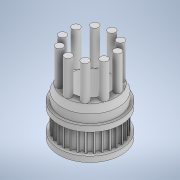
# Autodesk Inventor part: piece_roue_test_8
Saved by Autodesk Inventor 2020.1 (Build 241239000, 239)
## iProperties
Created: 2019-07-25
Part Number: piece_roue_test_8
Material: Générique
Document SubType Name: Modeling
Designer: marlo
Density: 1 g/cm^3
Appearance: Par défaut
Author: marlo
Autodesk Inventor part; units mm, degrees
ref_plane "YZ Plane" through (0, 0, 0) normal (1, 0, 0) x (0, 1, 0)
ref_plane "XZ Plane" through (0, 0, 0) normal (0, 1, 0) x (-1, 0, 0)
ref_plane "XY Plane" through (0, 0, 0) normal (0, 0, 1) x (1, 0, 0)
sketch "Esquisse2" plane through (0, 0, 0) normal (0, 1, 0) x (-1, 0, 0)
  circle A0 centre (0, 0) radius 18.5
  circle A1 centre (0, 0) radius 13.1
  dimension "d0" = 37
  dimension "d1" = 26.2
  constraints: 2 centre point, 2 coincident
  measures "d0" diameter of A0
  measures "d1" diameter of A1
extrude "Extrusion1" add sketch "Esquisse2" against normal blind 13
sketch "Esquisse3" plane through (0, 0, 0) normal (0, 1, 0) x (1, 0, 0)
  circle A0 centre (0, -15.8) radius 2.7
  line L0 (-22, 0) -> (25, 0) construction
  line L1 (-20, -18.5) -> (14, -18.5) construction
  circle A1 centre (0, 0) radius 18.5 construction
  circle A2 centre (-15.0267, 4.8825) radius 2.7
  line L2 (0, -15.8) -> (0, 0) construction
  line L3 (-15.0267, 4.8825) -> (0, 0) construction
  circle A3 centre (-15.0267, -4.8825) radius 2.7
  line L4 (0, 0) -> (-15.0267, -4.8825) construction
  line L5 (-15.0267, -4.8825) -> (-15.0267, 4.8825) construction
  line L6 (0, -31) -> (0, 24) construction
  line L7 (-15.0267, -4.8825) -> (-15.0267, -7.5825) construction
  line L8 (-15.0267, 4.8825) -> (-16.4693, 2.6002) construction
  line L9 (0, -15.8) -> (-2.3383, -17.15) construction
  circle A4 centre (-9.287, 12.7825) radius 2.7
  line L10 (0, 0) -> (-9.287, 12.7825) construction
  line L11 (-9.287, 12.7825) -> (-15.0267, 4.8825) construction
  line L12 (-9.287, 12.7825) -> (-7.7, 14.9668) construction
  circle A5 centre (-9.287, -12.7825) radius 2.7
  line L13 (-9.287, -12.7825) -> (0, 0) construction
  line L14 (-9.287, -12.7825) -> (0, -15.8) construction
  line L15 (-9.287, -12.7825) -> (-11.2119, -10.8891) construction
  line L16 (-9.287, -12.7825) -> (-15.0267, -4.8825) construction
  circle A6 centre (0, 15.8) radius 2.7
  line L17 (0, 15.8) -> (-1.5986, 17.9759) construction
  line L18 (0, 15.8) -> (0, 0) construction
  line L19 (0, 15.8) -> (-9.287, 12.7825) construction
  circle A7 centre (15.0267, 4.8825) radius 2.7
  circle A8 centre (15.0267, -4.8825) radius 2.7
  circle A9 centre (9.287, 12.7825) radius 2.7
  circle A10 centre (9.287, -12.7825) radius 2.7
  dimension "d4" = 5.4
  constraints: 40 end point, 14 equal length, 4 centre point, 4 symmetric about line, 3 horizontal, 3 point on line, 3 vertical, 1 coincident, 1 tangent, 1 vertical alignment, 21 other
extrude "Extrusion2" add sketch "Esquisse3" along normal blind 25
sketch "Esquisse4" plane through (0, -13, 0) normal (0, -1, 0) x (1, 0, 0)
  circle A0 centre (0, 0) radius 20.5
  circle A1 centre (0, 0) radius 13.1 projected
  circle A2 centre (0, 0) radius 18.5 projected
  circle A3 centre (0, 0) radius 13.1
  dimension "d9" = 2
  constraints: 2 centre point, 2 concentric, 1 coincident
  measures "d9" radial gap between concentric circles of A2 A0
extrude "Extrusion3" add sketch "Esquisse4" along normal blind 19 contours A0 | A2
sketch "Esquisse6" plane through (0, -13, 0) normal (0, 1, 0) x (1, 0, 0)
  line L0 (1.7624, -20.4241) -> (1.7106, -19.8241)
  line L1 (4.9624, -19.8903) -> (4.8166, -19.306)
  arc A0 (4.8166, -19.306) -> (1.7106, -19.8241) centre (3.2636, -19.5651) ccw
  arc A1 (1.7624, -20.4241) -> (4.9624, -19.8903) centre (0, 0) ccw
  circle A2 centre (0, 0) radius 20.5 projected
  line L2 (0, 0) -> (1.6349, -26.9944)
  line L3 (0.7154, -20.4875) -> (0.6944, -19.8857)
  line L4 (-2.5257, -20.3438) -> (-2.4515, -19.7462)
  arc A3 (0.6944, -19.8857) -> (-2.4515, -19.7462) centre (-0.8786, -19.8159) ccw
  arc A4 (-2.5257, -20.3438) -> (0.7154, -20.4875) centre (0, 0) ccw
  line L5 (0, 0) -> (0, -51.6999) construction
  line L6 (0.7154, -20.4875) -> (1.7624, -20.4241) construction
  line L7 (0, 0) -> (-3.8017, -25.3081)
  line L8 (-7.6853, -19.0049) -> (-7.4595, -18.4466)
  line L9 (-10.5872, -17.5545) -> (-10.2762, -17.0388)
  arc A5 (-7.4595, -18.4466) -> (-10.2762, -17.0388) centre (-8.8679, -17.7427) ccw
  arc A6 (-10.5872, -17.5545) -> (-7.6853, -19.0049) centre (0, 0) ccw
  line L10 (-6.7031, -19.3731) -> (-6.5062, -18.804)
  line L11 (-3.5629, -20.188) -> (-3.4583, -19.5949)
  arc A7 (-3.4583, -19.5949) -> (-6.5062, -18.804) centre (-4.9822, -19.1995) ccw
  arc A8 (-6.7031, -19.3731) -> (-3.5629, -20.188) centre (0, 0) ccw
  line L12 (-3.5629, -20.188) -> (-2.5257, -20.3438) construction
  line L13 (0, 0) -> (-19.3122, -30.2436)
  line L14 (-19.2701, -6.9937) -> (-18.704, -6.7882)
  line L15 (-20.1321, -3.8661) -> (-19.5407, -3.7525)
  arc A9 (-18.704, -6.7882) -> (-19.5407, -3.7525) centre (-19.1224, -5.2704) ccw
  arc A10 (-20.1321, -3.8661) -> (-19.2701, -6.9937) centre (0, 0) ccw
  line L16 (-18.8872, -7.9702) -> (-18.3323, -7.7361)
  line L17 (-17.3933, -10.85) -> (-16.8824, -10.5313)
  arc A11 (-16.8824, -10.5313) -> (-18.3323, -7.7361) centre (-17.6073, -9.1337) ccw
  arc A12 (-18.8872, -7.9702) -> (-17.3933, -10.85) centre (0, 0) ccw
  line L18 (-18.8872, -7.9702) -> (-19.2701, -6.9937) construction
  line L19 (-14.008, -14.9675) -> (-13.5964, -14.5278)
  line L20 (-11.4713, -16.99) -> (-11.1343, -16.4909)
  line L21 (-14.7552, -14.2314) -> (-14.3217, -13.8134)
  arc A13 (-11.1343, -16.4909) -> (-13.5964, -14.5278) centre (-12.3654, -15.5093) ccw
  arc A14 (-14.008, -14.9675) -> (-11.4713, -16.99) centre (0, 0) ccw
  arc A15 (-14.3217, -13.8134) -> (-16.3216, -11.381) centre (-15.3217, -12.5972) ccw
  line L22 (-16.8156, -11.7255) -> (-16.3216, -11.381)
  arc A16 (-16.8156, -11.7255) -> (-14.7552, -14.2314) centre (0, 0) ccw
  line L23 (-16.8156, -11.7255) -> (-17.3933, -10.85) construction
  line L24 (-11.4713, -16.99) -> (-10.5872, -17.5545) construction
  line L25 (0, 0) -> (-31.9499, -5.2919)
  line L26 (-4.9168, 19.9016) -> (-4.7723, 19.317)
  line L27 (-1.7156, 20.4281) -> (-1.6652, 19.828)
  arc A17 (-4.7723, 19.317) -> (-1.6652, 19.828) centre (-3.2187, 19.5725) ccw
  arc A18 (-1.7156, 20.4281) -> (-4.9168, 19.9016) centre (0, 0) ccw
  line L28 (-5.9283, 19.6241) -> (-5.7542, 19.0476)
  line L29 (-8.9499, 18.4431) -> (-8.687, 17.9013)
  arc A19 (-8.687, 17.9013) -> (-5.7542, 19.0476) centre (-7.2206, 18.4745) ccw
  arc A20 (-5.9283, 19.6241) -> (-8.9499, 18.4431) centre (0, 0) ccw
  line L30 (-5.9283, 19.6241) -> (-4.9168, 19.9016) construction
  line L31 (-13.4024, 15.5121) -> (-13.0086, 15.0564)
  line L32 (-15.6817, 13.2036) -> (-15.221, 12.8157)
  line L33 (-12.5914, 16.1774) -> (-12.2215, 15.7021)
  arc A21 (-15.221, 12.8157) -> (-13.0086, 15.0564) centre (-14.1148, 13.9361) ccw
  arc A22 (-13.4024, 15.5121) -> (-15.6817, 13.2036) centre (0, 0) ccw
  arc A23 (-12.2215, 15.7021) -> (-9.5913, 17.4335) centre (-10.9064, 16.5678) ccw
  line L34 (-9.8816, 17.9612) -> (-9.5913, 17.4335)
  arc A24 (-9.8816, 17.9612) -> (-12.5914, 16.1774) centre (0, 0) ccw
  line L35 (-9.8816, 17.9612) -> (-8.9499, 18.4431) construction
  line L36 (-20.496, 0.4072) -> (-19.8938, 0.3953)
  line L37 (-20.3035, -2.8313) -> (-19.7071, -2.7481)
  arc A25 (-19.7071, -2.7481) -> (-19.8938, 0.3953) centre (-19.8005, -1.1764) ccw
  arc A26 (-20.496, 0.4072) -> (-20.3035, -2.8313) centre (0, 0) ccw
  line L38 (-18.0857, 9.6519) -> (-17.5544, 9.3683)
  arc A27 (-17.5544, 9.3683) -> (-15.8566, 12.0204) centre (-16.7055, 10.6943) ccw
  arc A28 (-16.3365, 12.3842) -> (-18.0857, 9.6519) centre (0, 0) ccw
  line L39 (-16.3365, 12.3842) -> (-15.8566, 12.0204)
  line L40 (-20.4483, 1.4551) -> (-19.8476, 1.4123)
  line L41 (-19.9627, 4.6627) -> (-19.3762, 4.5258)
  line L42 (-18.5557, 8.7142) -> (-18.0106, 8.4582)
  arc A29 (-18.5557, 8.7142) -> (-19.6981, 5.6777) centre (0, 0) ccw
  arc A30 (-19.1194, 5.5109) -> (-18.0106, 8.4582) centre (-18.565, 6.9845) ccw
  line L43 (-19.6981, 5.6777) -> (-19.1194, 5.5109)
  line L44 (-19.6981, 5.6777) -> (-19.9627, 4.6627) construction
  arc A31 (-19.9627, 4.6627) -> (-20.4483, 1.4551) centre (0, 0) ccw
  arc A32 (-19.8476, 1.4123) -> (-19.3762, 4.5258) centre (-19.6119, 2.969) ccw
  line L45 (-20.4483, 1.4551) -> (-20.496, 0.4072) construction
  line L46 (-16.3365, 12.3842) -> (-15.6817, 13.2036) construction
  line L47 (-20.3035, -2.8313) -> (-20.1321, -3.8661) construction
  line L48 (0, 0) -> (-1.2679, 21.7616)
  line L49 (7.7288, 18.9872) -> (6.7475, 19.3577) construction
  arc A33 (7.5018, 18.4294) -> (10.3152, 17.0152) centre (8.9085, 17.7223) ccw
  arc A34 (10.6274, 17.5302) -> (7.7288, 18.9872) centre (0, 0) ccw
  line L50 (10.6274, 17.5302) -> (10.3152, 17.0152)
  line L51 (11.5102, 16.9636) -> (11.1721, 16.4653)
  line L52 (7.7288, 18.9872) -> (7.5018, 18.4294)
  line L53 (6.7475, 19.3577) -> (6.5493, 18.789)
  arc A35 (6.7475, 19.3577) -> (3.6092, 20.1798) centre (0, 0) ccw
  arc A36 (3.5032, 19.587) -> (6.5493, 18.789) centre (5.0262, 19.188) ccw
  line L54 (2.5723, 20.338) -> (2.4967, 19.7405)
  line L55 (-0.6684, 20.4891) -> (-0.6488, 19.8872)
  line L56 (14.7878, 14.1976) -> (14.0422, 14.9354) construction
  arc A37 (11.1721, 16.4653) -> (13.6297, 14.4966) centre (12.4009, 15.481) ccw
  line L57 (3.6092, 20.1798) -> (3.5032, 19.587)
  arc A38 (14.3534, 13.7805) -> (16.3476, 11.3436) centre (15.3505, 12.562) ccw
  arc A39 (16.8424, 11.6869) -> (14.7878, 14.1976) centre (0, 0) ccw
  arc A40 (14.0422, 14.9354) -> (11.5102, 16.9636) centre (0, 0) ccw
  line L58 (14.7878, 14.1976) -> (14.3534, 13.7805)
  line L59 (16.8424, 11.6869) -> (16.3476, 11.3436)
  line L60 (14.0422, 14.9354) -> (13.6297, 14.4966)
  arc A41 (-0.6488, 19.8872) -> (2.4967, 19.7405) centre (0.924, 19.8139) ccw
  arc A42 (2.5723, 20.338) -> (-0.6684, 20.4891) centre (0, 0) ccw
  arc A43 (20.141, 3.8199) -> (19.2861, 6.9495) centre (0, 0) ccw
  arc A44 (18.7195, 6.7454) -> (19.5493, 3.7077) centre (19.1344, 5.2265) ccw
  line L61 (20.141, 3.8199) -> (19.5493, 3.7077)
  line L62 (3.6092, 20.1798) -> (2.5723, 20.338) construction
  line L63 (18.9054, 7.9269) -> (18.35, 7.694)
  arc A45 (16.9064, 10.4925) -> (18.35, 7.694) centre (17.6282, 9.0933) ccw
  line L64 (17.4181, 10.8101) -> (16.9064, 10.4925)
  arc A46 (18.9054, 7.9269) -> (17.4181, 10.8101) centre (0, 0) ccw
  line L65 (19.2861, 6.9495) -> (18.7195, 6.7454)
  line L66 (-1.7156, 20.4281) -> (-0.6684, 20.4891) construction
  line L67 (0, 0) -> (10.297, 1.6813)
  line L68 (20.31, 2.7847) -> (19.7133, 2.7029)
  arc A47 (19.7133, 2.7029) -> (19.8929, -0.4409) centre (19.8031, 1.131) ccw
  arc A48 (20.495, -0.4542) -> (20.31, 2.7847) centre (0, 0) ccw
  line L69 (20.495, -0.4542) -> (19.8929, -0.4409)
  line L70 (20.31, 2.7847) -> (20.141, 3.8199) construction
  circle A49 centre (0, 0) radius 20.5
  line L71 (1.7106, -19.8241) -> (4.8166, -19.306) construction
  line L72 (0, 0) -> (36.3329, -1.736)
  line L73 (18.0635, -9.6933) -> (17.5329, -9.4085)
  arc A50 (17.5329, -9.4085) -> (15.829, -12.0567) centre (16.6809, -10.7326) ccw
  arc A51 (16.3081, -12.4216) -> (18.0635, -9.6933) centre (0, 0) ccw
  line L74 (16.3081, -12.4216) -> (15.829, -12.0567)
  line L75 (9.8404, -17.9838) -> (9.5513, -17.4555)
  arc A52 (12.1855, -15.7301) -> (9.5513, -17.4555) centre (10.8684, -16.5928) ccw
  arc A53 (9.8404, -17.9838) -> (12.5543, -16.2062) centre (0, 0) ccw
  line L76 (12.5543, -16.2062) -> (12.1855, -15.7301)
  line L77 (13.3668, -15.5428) -> (12.5543, -16.2062) construction
  arc A54 (15.1916, -12.8505) -> (12.9741, -15.0862) centre (14.0829, -13.9684) ccw
  line L78 (15.6514, -13.2395) -> (15.1916, -12.8505)
  arc A55 (13.3668, -15.5428) -> (15.6514, -13.2395) centre (0, 0) ccw
  line L79 (13.3668, -15.5428) -> (12.9741, -15.0862)
  line L80 (19.685, -5.7228) -> (19.1067, -5.5547)
  arc A56 (19.1067, -5.5547) -> (17.9911, -8.4994) centre (18.5489, -7.0271) ccw
  arc A57 (18.5357, -8.7567) -> (19.685, -5.7228) centre (0, 0) ccw
  line L81 (18.5357, -8.7567) -> (17.9911, -8.4994)
  line L82 (20.4449, -1.5019) -> (19.8443, -1.4578)
  arc A58 (19.8443, -1.4578) -> (19.3658, -4.5701) centre (19.6051, -3.014) ccw
  arc A59 (19.952, -4.7085) -> (20.4449, -1.5019) centre (0, 0) ccw
  line L83 (19.952, -4.7085) -> (19.3658, -4.5701)
  line L84 (20.4449, -1.5019) -> (20.495, -0.4542) construction
  line L85 (0, 0) -> (16.0028, -31.1104)
  arc A60 (5.8833, -19.6376) -> (8.9076, -18.4636) centre (0, 0) ccw
  line L86 (5.8833, -19.6376) -> (5.7105, -19.0607)
  arc A61 (8.646, -17.9212) -> (5.7105, -19.0607) centre (7.1782, -18.491) ccw
  line L87 (8.9076, -18.4636) -> (8.646, -17.9212)
  line L88 (8.9076, -18.4636) -> (9.8404, -17.9838) construction
  point P0 (0, -18.5)
  point P1 (-10.874, -14.9668)
  point P2 (2.2327, -18.3648)
  point P3 (-5.4354, -17.6835)
  point P4 (-7.5298, -16.8983)
  point P5 (-16.7832, -7.783)
  point P6 (-9.0031, -16.1615)
  point P7 (-17.5998, -5.7007)
  point P8 (-13.7557, -12.3705)
  point P9 (-12.1623, -13.9402)
  point P10 (-5.9647, 17.5121)
  point P11 (-15.1189, 10.6616)
  point P12 (-3.8077, 18.1039)
  point P13 (-10.8466, 14.9867)
  point P14 (-12.5759, 13.5682)
  point P15 (-18.3963, 1.9563)
  point P16 (-13.733, 12.3957)
  point P17 (-17.0096, 7.2749)
  point P18 (-18.4979, -0.2782)
  point P19 (-16.0073, 9.2745)
  point P20 (10.9151, 14.9369)
  point P21 (13.7784, 12.3453)
  point P22 (1.6794, 18.4236)
  point P23 (3.8906, 18.0863)
  point P24 (9.0327, 16.145)
  point P25 (16.0497, 9.201)
  point P26 (18.4051, 1.8719)
  point P27 (14.8219, 11.0707)
  point P28 (12.2006, 13.9067)
  point P29 (18.0446, 4.0794)
  point P30 (-0.0435, -19.6183)
  point P31 (0, -20.5)
  point P32 (6.7475, 19.3577)
  point P33 (3.6092, 20.1798)
  point P34 (-19.9627, 4.6627)
  point P35 (-20.4483, 1.4551)
  point P36 (18.1427, -3.6182)
  point P37 (15.0993, -10.6893)
  point P38 (17.5735, -5.7813)
  point P39 (19.685, -5.7228)
  point P40 (18.0635, -9.6933)
  point P41 (13.3668, -15.5428)
  point P42 (9.8404, -17.9838)
  point P43 (12.5543, -16.2062)
  point P44 (8.9076, -18.4636)
  dimension "d17" = 3.2
  dimension "d34" = 0.6
  dimension "d35" = 1.5744
  dimension "d36" = 1.047
  constraints: 178 end point, 178 symmetric about line, 121 point on circle, 61 centre point, 8 equal length, 5 coincident, 2 line through centre, 1 midpoint, 1 point on line, 1 vertical, 58 other
  measures "d17" horizontal distance of L1.start L0.start
  measures "d34" vertical distance of L0.start L0.end
  measures "d35" radius of A0
  measures "d36" horizontal distance of L3.start L0.start
extrude "Extrusion5" cut sketch "Esquisse6" against normal blind 17 contours L0 A0 L1 A1 | L86 A61 L87 A2 | A2 L4 A3 L3 | A2 L10 A7 L11 | A2 L19 A13 L20 | L9 A5 L8 A2 | A2 L36 A25 L37 | L15 A9 L14 A2 | A2 L54 A41 L55 | L27 A17 L26 A2 | A2 L83 A58 L82 | L69 A47 L68 A2 | L75 A52 L76 A2 | A2 L22 A15 L21 | A2 L41 A32 L40 | L16 A11 L17 A2 | A2 L53 A36 L57 | L28 A19 L29 A2 | A2 L81 A56 L80 | L79 A54 L78 A2 | L61 A44 L65 A2 | A2 L42 A30 L43 | A2 L50 A33 L52 | L34 A23 L33 A2 | A2 L74 A50 L73 | L63 A45 L64 A2 | A2 L39 A27 L38 | A2 L60 A37 L51 | L31 A21 L32 A2 | L59 A38 L58 A2
sketch "Esquisse7" plane through (0, -32, 0) normal (0, -1, 0) x (1, 0, 0)
  circle A0 centre (0, 0) radius 20.5 projected
  circle A1 centre (0, 0) radius 20.5
  circle A2 centre (0, 0) radius 13.1
  point P0 (20.5, 0)
  point P1 (20.5, 0)
  point P2 (20.5, 0)
  point P3 (-3.2, 20.2487)
  point P4 (20.5, 0)
  point P5 (20.494, -0.4946)
  point P6 (20.4248, 1.7546)
  point P7 (20.4248, 1.7546)
  point P8 (20.5, 0)
  point P9 (19.64, -5.8755)
  constraints: 2 centre point, 2 coincident, 1 point on circle
extrude "Extrusion6" add sketch "Esquisse7" along normal blind 2
sketch "Esquisse8" plane through (0, 0, 0) normal (0, 1, 0) x (1, 0, 0)
  arc A0 (-8.887, -16.2257) -> (-7.0807, -17.0913) centre (0, 0) ccw projected
  circle A1 centre (0, 0) radius 18.5
  arc A2 (19.9005, -4.9213) -> (20.4248, -1.7546) centre (0, 0) ccw projected
  circle A3 centre (0, 0) radius 20.5
  point P0 (-7.8462, -18.939)
  point P1 (-9.6565, -18.0832)
  point P2 (-8.887, -16.2257)
  point P3 (-7.8462, -18.939)
  point P4 (-9.6565, -18.0832)
  point P5 (-3.2, -20.2487)
  point P6 (0, -20.5)
  constraints: 2 coincident, 1 centre point, 3 other
extrude "Extrusion7" add sketch "Esquisse8" against normal blind 15
chamfer "Chanfrein2" distance 2 distance2 5 2 edges at (-20.2247, 0, -3.3482) (20.2247, 0, 3.3482) measured on face at (19.7314, 0, 3.2666) measured on face at (-19.7314, 0, -3.2666)
sketch "Esquisse9" plane through (0, -34, 0) normal (0, -1, 0) x (1, 0, 0)
  circle A0 centre (0, 0) radius 22.5
  circle A1 centre (0, 0) radius 20.5 projected
  circle A2 centre (0, 0) radius 20.5
  dimension "d39" = 2
  constraints: 2 centre point, 2 coincident
  measures "d39" radial gap between concentric circles of A0 A1
extrude "Extrusion8" add sketch "Esquisse9" against normal blind 4
sketch "Esquisse10" plane through (0, -15, 0) normal (0, -1, 0) x (1, 0, 0)
  circle A0 centre (0, 0) radius 22.5
  circle A1 centre (0, 0) radius 22.5 projected
  circle A2 centre (0, 0) radius 20.5
  constraints: 2 centre point, 2 coincident
extrude "Extrusion9" add sketch "Esquisse10" against normal blind 4
